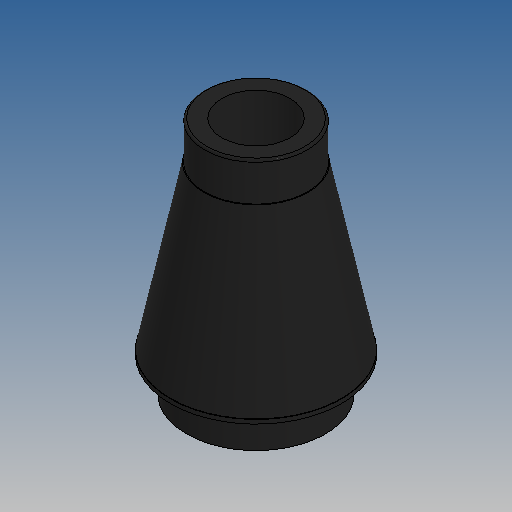
# Autodesk Inventor part: 59900-Black
Saved by Autodesk Inventor 2025.1 (Build 291241000, 241)
## iProperties
Created: 2014-06-03
Part Number: 59900-Black
Material: ABS Plastic
Document SubType Name: Modeling
Designer: D. Kohfeld
Density: 1.06 g/cm^3
Appearance: Black
Mass: 0.246098 g
Surface Area: 4.12115 cm^2
Volume: 0.232168 cm^3
Author: D. Kohfeld
Autodesk Inventor part; units mm, degrees
ref_plane "YZ Plane" through (0, 0, 0) normal (1, 0, 0) x (0, 1, 0)
ref_plane "XZ Plane" through (0, 0, 0) normal (0, 1, 0) x (-1, 0, 0)
ref_plane "XY Plane" through (0, 0, 0) normal (0, 0, 1) x (1, 0, 0)
sketch "Sketch11" plane through (0, 0, 0) normal (1, 0, 0) x (0, 1, 0)
  line L0 (0, 3.2569) -> (1.6, 3.2569)
  line L1 (1.6, 4) -> (1.8, 4)
  line L2 (-2.24, 0) -> (13.44, 0) projected
  line L3 (1.6, 3.2569) -> (1.6, 4)
  line L4 (1.8, 4) -> (9.6, 2.4)
  line L5 (9.6, 2.4) -> (11.2, 2.4)
  line L6 (11.2, 2.4) -> (11.2, 1.6)
  line L7 (11.2, 1.6) -> (3.6, 1.6)
  line L8 (3.6, 1.6) -> (3.6, 2.4)
  line L9 (3.6, 2.4) -> (0, 2.4)
  line L10 (0, 2.4) -> (0, 3.2569)
  line L11 (9.6, 2.4) -> (9.4, 2.4)
  line L12 (9.4, 2.4) -> (9.4, 2.441)
  point P0 (0, 0)
  dimension "d99" = 4.8
  dimension "d100" = 1.6
  dimension "d101" = 6.5137
  dimension "d102" = 8
  dimension "d104" = 3.2
  dimension "d105" = 4.8
  dimension "d106" = 1.6
  dimension "d107" = 9.6
  dimension "d109" = 3.6
  dimension "d110" = 0.2
  dimension "d116" = 1.8
  constraints: 24 end point, 8 perpendicular, 1 point on line, 1 vertical, 1 vertical alignment
  measures "d99" diameter of L9 L2
  measures "d100" distance between parallel lines of L3 L10
  measures "d101" diameter of L0 L2
  measures "d102" diameter of L1 L2
  measures "d104" diameter of L7 L2
  measures "d105" diameter of L5 L2
  measures "d106" distance from line of L4.end L6
  measures "d107" distance from line of L4.end L10
  measures "d109" distance between parallel lines of L8 L10
  measures "d110" distance from line of L1.end L3
  measures "d116" distance between parallel lines of L6 L12
revolve "Revolution1" add sketch "Sketch11" angle 360 about axis through (0, -10, 0) along (0, 1, 0) contours L0 L3 L1 L4 L12 L11 L5 L6 L7 L8 L9 L10
fillet "Fillet1" radius 0.1 2 edges at (0, 11.2, -2.4) (0, 1.8, -4)
sketch "Sketch12" plane through (0, 3.6, 0) normal (0, -1, 0) x (1, 0, 0)
  circle A0 centre (0, 0) radius 2.4 projected
  line L0 (-0.8, 2.2627) -> (-0.8, 0.8)
  line L1 (-0.8, 0.8) -> (-2.2627, 0.8)
  line L2 (-2.2627, -0.8) -> (-0.8, -0.8)
  line L3 (-0.8, -0.8) -> (-0.8, -2.2627)
  line L4 (0.8, -2.2627) -> (0.8, -0.8)
  line L5 (0.8, -0.8) -> (2.2627, -0.8)
  line L6 (2.2627, 0.8) -> (0.8, 0.8)
  line L7 (0.8, 0.8) -> (0.8, 2.2627)
  dimension "d111" = 1.6
  constraints: 16 end point, 7 equal length, 4 perpendicular, 3 parallel, 1 vertical, 9 other
  measures "d111" distance between parallel lines of L7 L0
extrude "Extrusion7" add sketch "Sketch12" along normal blind 1.8 contours L6 L7 A0 | A0 L4 L5 | L0 L1 A0 | A0 L2 L3
equation "\"d99\" = kd"
equation "\"d100\" = 0.333333 * lh - topthk"
equation "\"d101\" = tubeod"
equation "\"d102\" = lu"
equation "\"d104\" = rd"
equation "\"d105\" = kd"
equation "\"d106\" = knobh"
equation "\"d107\" = lh"
equation "\"d22\" = lf"
equation "\"d111\" = axlet"
equation "\"kd\" = 4.8"
equation "\"lh\" = 9.6"
equation "\"topthk\" = 1.6"
equation "\"tubeod\" = 6.513708"
equation "\"lu\" = 8"
equation "\"rd\" = 3.2"
equation "\"knobh\" = 1.6"
equation "\"lf\" = 0.1"
equation "\"axlet\" = 1.6"
body "Solid1"
body "Solid2"
